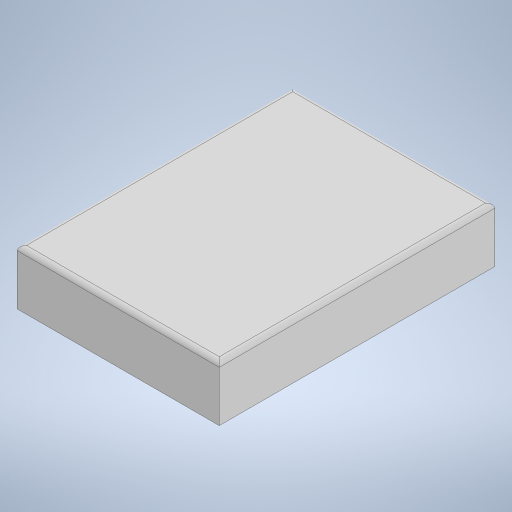
# Autodesk Inventor part: phan1_cuaTrung
Saved by Autodesk Inventor 2023 (Build 270158000, 158)
## iProperties
Created: 2022-11-20
Part Number: phan1_cuaTrung
Material: Generic
Document SubType Name: Modeling
Designer: ADMIN
Density: 1 g/cm^3
Appearance: Default
Author: ADMIN
Autodesk Inventor part; units mm, degrees
ref_plane "YZ Plane" through (0, 0, 0) normal (1, 0, 0) x (0, 1, 0)
ref_plane "XZ Plane" through (0, 0, 0) normal (0, 1, 0) x (-1, 0, 0)
ref_plane "XY Plane" through (0, 0, 0) normal (0, 0, 1) x (1, 0, 0)
sketch "Sketch1" plane through (0, 0, 0) normal (0, 1, 0) x (-1, 0, 0)
  line L0 (10.8236, 13.6023) -> (-209.1764, 13.6023)
  line L1 (-209.1764, 13.6023) -> (-209.1764, -286.3977)
  line L2 (-209.1764, -286.3977) -> (10.8236, -286.3977)
  line L3 (10.8236, -286.3977) -> (10.8236, 13.6023)
  point P0 (0, 0)
  dimension "d0" = 220
  dimension "d1" = 300
  constraints: 8 end point, 2 parallel, 1 horizontal, 1 perpendicular
  measures "d0" distance of L2.end L1.end
  measures "d1" distance of L1.end L0.end
extrude "Extrusion1" add sketch "Sketch1" along normal blind 60
fillet "Fillet1" radius 5 1 edges at (209.1764, 60, -136.3977)
fillet "Fillet1" radius 5 1 edges at (99.1764, 60, 13.6023)
fillet "Fillet1" radius 5 1 edges at (-10.8236, 60, -136.3977)
fillet "Fillet1" radius 5 1 edges at (99.1764, 60, -286.3977)
body "Solid1"
